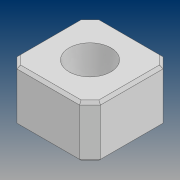
# Autodesk Inventor part: Vong_chan
Saved by Autodesk Inventor 2021 (Build 250183000, 183)
## iProperties
Created: 2024-04-08
Part Number: Vong_chan
Material: Generic
Document SubType Name: Modeling
Designer: Admin
Density: 1 g/cm^3
Appearance: Default
Author: Admin
Autodesk Inventor part; units mm, degrees
ref_plane "YZ Plane" through (0, 0, 0) normal (1, 0, 0) x (0, 1, 0)
ref_plane "XZ Plane" through (0, 0, 0) normal (0, 1, 0) x (-1, 0, 0)
ref_plane "XY Plane" through (0, 0, 0) normal (0, 0, 1) x (1, 0, 0)
sketch "Sketch1" plane through (0, 0, 0) normal (0, 1, 0) x (-1, 0, 0)
  line L0 (-8, 8) -> (-8, -8)
  line L1 (-8, -8) -> (8, -8)
  line L2 (8, -8) -> (8, 8)
  line L3 (8, 8) -> (-8, 8)
  line L4 (-8, 8) -> (8, -8) construction
  line L5 (-8, -8) -> (8, 8) construction
  circle A0 centre (0, 0) radius 4
  dimension "d0" = 16
  dimension "d1" = 8
  constraints: 12 end point, 2 midpoint, 2 parallel, 2 perpendicular, 1 centre point, 1 coincident, 1 vertical
  measures "d0" distance of L0.end L1.end
  measures "d1" diameter of A0
extrude "Extrusion1" add sketch "Sketch1" along normal mid plane 10
chamfer "Chamfer1" distance 2 angle 45 4 edges at (8, 0, 8) (8, 0, -8) (-8, 0, 8) (-8, 0, -8)
chamfer "Chamfer2" distance 0.5 angle 45 16 edges at (-8, -5, 0) (-7, -5, -7) (0, -5, -8) (8, -5, 0) (7, -5, 7) (0, -5, 8) (-7, -5, 7) (7, -5, -7) (-7, 5, 7) (0, 5, 8) (-8, 5, 0) (-7, 5, -7) (0, 5, -8) (7, 5, -7) (8, 5, 0) (7, 5, 7)
body "Solid1"
